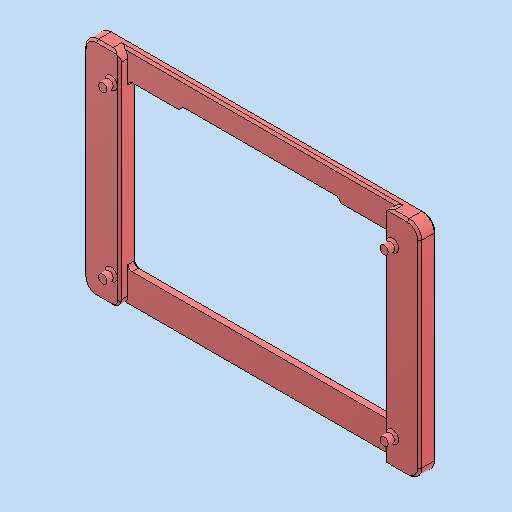
# Autodesk Inventor part: screen-frame
Saved by Autodesk Inventor 2026 (Build 300175050, 175E)
## iProperties
Created: 2025-06-21
Part Number: screen-frame
Material: ABS Plastic
Document SubType Name: Modeling
Designer: queezz
Density: 1.06 g/cm^3
Appearance: Smooth - Red
Author: queezz
Autodesk Inventor part; units mm, degrees
ref_plane "YZ Plane" through (0, 0, 0) normal (1, 0, 0) x (0, 1, 0)
ref_plane "XZ Plane" through (0, 0, 0) normal (0, 1, 0) x (-1, 0, 0)
ref_plane "XY Plane" through (0, 0, 0) normal (0, 0, 1) x (1, 0, 0)
sketch "Sketch1" plane through (0, 0, 0) normal (0, 0, 1) x (1, 0, 0)
  line L0 (-40, 26.5) -> (40, 26.5)
  line L1 (40, 26.5) -> (40, -26.5)
  line L2 (40, -26.5) -> (-40, -26.5)
  line L3 (-40, -26.5) -> (-40, 26.5)
  line L4 (31.5, 20) -> (-31.5, 20)
  line L5 (-31.5, 20) -> (-31.5, -19)
  line L6 (-31.5, -19) -> (31.5, -19)
  line L7 (31.5, -19) -> (31.5, 20)
  line L8 (-19, 20) -> (19, 20)
  line L9 (19, 20) -> (19, 21)
  line L10 (19, 21) -> (-19, 21)
  line L11 (-19, 21) -> (-19, 20)
  line L12 (-33.5, 19.5) -> (33.5, 19.5) construction
  line L13 (33.5, 19.5) -> (33.5, -20) construction
  line L14 (33.5, -20) -> (-33.5, -20) construction
  line L15 (-33.5, -20) -> (-33.5, 19.5) construction
  line L16 (-31.5, 20) -> (-31.5, 26.5)
  line L17 (-31.5, -19) -> (-31.5, -26.5)
  line L18 (31.5, -19) -> (31.5, -26.5)
  line L19 (31.5, 20) -> (31.5, 26.5)
  point P0 (0, 0)
  point P1 (40, 0)
  point P2 (0, 26.5)
  point P3 (31.5, 0.5)
  point P4 (0, 20)
  point P5 (0, -20)
  dimension "d0" = 53
  dimension "d1" = 80
  dimension "d30" = 63
  dimension "d32" = 38
  dimension "d33" = 1
  dimension "d34" = 67
  dimension "d35" = 39.5
  dimension "d46" = 19.5
  dimension "d52" = 20
  dimension "d53" = 19
  constraints: 40 end point, 8 parallel, 8 point on line, 6 midpoint, 5 perpendicular, 4 coincident, 4 horizontal, 3 vertical alignment, 1 horizontal alignment
  measures "d0" distance of L0.end L1.end
  measures "d1" distance of L0.start L0.end
  measures "d30" distance of L5.end L6.end
  measures "d32" distance of L9.end L10.end
  measures "d33" distance of L8.end L9.end
  measures "d34" distance of L13.end L14.end
  measures "d35" distance of L14.end L12.start
  measures "d46" distance from line of point (0, 0) L12
  measures "d52" distance from line of point (0, 0) L4
  measures "d53" distance from line of L6 point (0, 0)
extrude "Extrusion1" add sketch "Sketch1" against normal blind 2 contours L0 L16 L5 L17 L2 L3 | L0 L19 L4 L9 L10 L11 L16 | L0 L1 L2 L18 L7 L19 | L17 L6 L18 L2
extrude "Extrusion5" add sketch "Sketch1" along normal blind 2 contours L0 L16 L5 L17 L2 L3 | L0 L1 L2 L18 L7 L19
sketch "Sketch6" plane through (0, 0, 2) normal (0, 0, 1) x (1, 0, 0)
  circle A0 centre (-33.5, 19.5) radius 1
  circle A1 centre (33.5, 19.5) radius 1
  circle A2 centre (33.5, -20) radius 1
  circle A3 centre (-33.5, -20) radius 1
  point P0 (0, 0)
  dimension "d40" = 2
  constraints: 4 centre point, 4 coincident, 3 equal radius
  measures "d40" diameter of A0
extrude "Extrusion6" add sketch "Sketch6" along normal blind 2
fillet "Fillet3" radius 1 8 edges at (19, 20, -1) (19, 21, -1) (-19, 20, -1) (-19, 21, -1) (-31.5, 20, -1) (31.5, 20, -1) (31.5, -19, -1) (-31.5, -19, -1)
fillet "Fillet4" radius 3 4 edges at (40, -26.5, 0) (-40, -26.5, 0) (-40, 26.5, 0) (40, 26.5, 0)
chamfer "Chamfer2" distance 0.5 angle 45 40 edges at (-31.5, 0, 2) (-34.5, 19.5, 2) (-34.5, -20, 2) (31.5, 0, 2) (32.5, 19.5, 2) (32.5, -20, 2) (34.25, -26.5, 2) (39.1213, -25.6213, 2) (40, 0, 2) (39.1213, 25.6213, 2) (34.25, 26.5, 2) (-39.1213, -25.6213, 2) (-40, 0, 2) (-39.1213, 25.6213, 2) (-34.25, 26.5, 2) (-34.25, -26.5, 2) (0, -26.5, -2) (-39.1213, -25.6213, -2) (-40, 0, -2) (-39.1213, 25.6213, -2) (0, 26.5, -2) (39.1213, 25.6213, -2) (40, 0, -2) (39.1213, -25.6213, -2) (0, 21, -2) (-18.5001, 20.866, -2) (-19.2321, 20.134, -2) (-25.1161, 20, -2) (-31.2071, 19.7071, -2) (-31.5, 0.5, -2) (-31.2071, -18.7071, -2) (0, -19, -2) (31.2071, -18.7071, -2) (31.5, 0.5, -2) (31.2071, 19.7071, -2) (25.1161, 20, -2) (19.2321, 20.134, -2) (18.5001, 20.866, -2) (0, 26.5, 0) (0, -26.5, 0)
fillet "Fillet5" radius 2 9 edges at (-31.5, 26.5, 0.75) (-31.5, 26.5, -0.25) (31.5, 26.5, 0.75) (31.5, 26.5, -0.25) (31.5, -26.5, 0.75) (31.5, -26.5, -0.25) (-31.75, -26.25, 1.7501) (-31.5, -26.5, 0.75) (-31.5, -26.5, -0.25)
equation "\"d40\" = peg"
equation "\"shift\" = 0.5"
equation "\"peg\" = 2"
body "Solid1"
